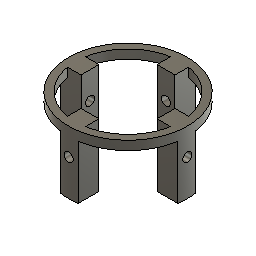
Nema17_Motor_mount_coupling_Part2 (Autodesk Fusion 360 design; units mm, degrees)
part number: 2025-04-23-20-16-13-902
Autodesk Fusion 360 part; units mm, degrees
sketch "Sketch1" plane through (0, 0, 0) normal (0, 1, 0) x (1, 0, 0)
  circle A0 centre (0, 0) radius 11
  circle A1 centre (0, 0) radius 20
  line L0 (0, 0) -> (25.4951, 0) construction
  circle A2 centre (10, 10) radius 1.5
  circle A3 centre (-10, 10) radius 1.5
  circle A4 centre (-10, -10) radius 1.5
  circle A5 centre (10, -10) radius 1.5
  dimension "d1" = 22
  dimension "d2" = 40
  dimension "d4" = 3
  dimension "d5" = 10
  dimension "d7" = 360
  constraint coincident A0.centre A1.centre
  constraint concentric A0 A1
  constraint horizontal L0
  measures "d1" diameter of A0
  measures "d2" diameter of A1
  measures "d4" diameter of A2
  measures "d5" horizontal distance of A0.centre A2.centre
extrude "Extrude1" add sketch "Sketch1" along normal blind 2
sketch "Sketch2" plane through (0, 2, 0) normal (0, 1, 0) x (-1, 0, 0)
  circle A0 centre (10, 10) radius 1.5
  circle A1 centre (10, -10) radius 1.5
  circle A2 centre (-10, -10) radius 1.5
  circle A3 centre (0, 0) radius 11
  circle A4 centre (-10, 10) radius 1.5
  circle A5 centre (0, 0) radius 20
  circle A6 centre (0, 0) radius 18
  circle A7 centre (0, 0) radius 20
  dimension "d10" = 36
  constraint concentric A3 A6
  constraint concentric A3 A7
  measures "d10" diameter of A6
extrude "Extrude2" add sketch "Sketch2" along normal blind 30 contours A5 A7
sketch "Sketch7" plane through (0, 32, 0) normal (0, 1, 0) x (-1, 0, 0)
  circle A0 centre (0, 0) radius 18
  circle A1 centre (0, 0) radius 20
  circle A2 centre (0, 0) radius 33.1
  circle A3 centre (0, 0) radius 20
  dimension "d24" = 66.2
  constraint concentric A0 A2
  constraint coincident A0.centre A1.centre
  measures "d24" diameter of A2
extrude "Extrude6" add sketch "Sketch7" against normal blind 4 contours A2
sketch "Sketch8" plane through (0, 28, 0) normal (0, -1, 0) x (1, 0, 0)
  circle A0 centre (0, 0) radius 20
  circle A1 centre (0, 0) radius 33.1
  circle A2 centre (0, 0) radius 22.5
  dimension "d31" = 45
  constraint coincident A0.centre A1.centre
  measures "d31" diameter of A2
extrude "Extrude7" add sketch "Sketch8" along normal blind 8 contours A2
sketch "Sketch9" plane through (0, 32, 0) normal (0, 1, 0) x (-1, 0, 0)
  circle A0 centre (0, 0) radius 33.1
  circle A1 centre (0, 0) radius 18
  circle A2 centre (0, 0) radius 33.1
  circle A3 centre (0, 0) radius 29.1
  line L0 (21.15, -21.15) -> (-21.15, 21.15) construction
  line L1 (-21.15, -21.15) -> (21.15, 21.15) construction
  line L2 (-5, -21.15) -> (5, -21.15)
  line L3 (5, -21.15) -> (5, -32.7202)
  line L4 (-5, -32.7202) -> (-5, -21.15)
  line L5 (-5, -21.15) -> (3.5808, -32.9057) construction
  line L6 (5, -21.15) -> (-3.5808, -32.9057) construction
  line L7 (32.7202, -5) -> (21.15, -5)
  line L8 (21.15, 5) -> (32.7202, 5)
  line L9 (21.15, -5) -> (21.15, 5)
  line L10 (5, 32.7202) -> (5, 21.15)
  line L11 (-5, 21.15) -> (-5, 32.7202)
  line L12 (5, 21.15) -> (-5, 21.15)
  line L13 (-32.7202, 5) -> (-21.15, 5)
  line L14 (-21.15, -5) -> (-32.7202, -5)
  line L15 (-21.15, 5) -> (-21.15, -5)
  point P0 (0, -28)
  dimension "d34" = 4
  dimension "d35" = 42.3
  dimension "d36" = 42.3
  constraint coincident A0.centre A1.centre
  constraint coincident L0 A0.centre
  constraint coincident L1 A0.centre
  constraint horizontal L2
  constraint perpendicular L2 L3
  constraint parallel L3 L4
  constraint coincident L5 P0
  constraint coincident L6 P0
  constraint coincident A0 L3.end
  constraint coincident A0 L4.start
  constraint coincident A0 L6.end
  constraint coincident A0 L5.end
  constraint coincident A0 L14.end
  constraint coincident A0 L13.start
  constraint coincident A0 L11.end
  constraint coincident A0 L10.start
  constraint coincident A0 L7.start
  constraint coincident A0 L8.end
  measures "d34" distance of A2 A3
  measures "d35" distance of L0.end L1.end
  measures "d36" distance of L1.start L0.end
extrude "Extrude8" add sketch "Sketch9" along normal blind 35 contours A0 A2 A3 L7 L8 | A0 A2 A3 L10 L11 | A3 L7 L8 L9 | A0 A2 A3 L3 L4 | A3 L10 L11 L12 | A3 L2 L3 L4 | A0 A2 A3 L13 L14 | A3 L13 L14 L15
extrude "Extrude9" add sketch "Sketch9" along normal blind 5 from surface at 30 contours A0 A2 A3 L8 L10 | A0 A2 A3 L3 L7 | A0 A2 A3 L11 L13 | A0 A2 A3 L4 L14
sketch "Sketch10" plane through (0, 0, 0) normal (0, 0, 1) x (1, 0, 0)
  circle A0 centre (0, 52) radius 2.5
  line L0 (33.1, 67) -> (-33.1, 67)
  line L1 (-33.1, 28) -> (33.1, 28)
  dimension "d45" = 5
  dimension "d56" = 24
  measures "d45" diameter of A0
  measures "d56" distance of A0.centre L1
extrude "Extrude10" cut sketch "Sketch10" along normal mid plane 88
sketch "Sketch11" plane through (0, 0, 0) normal (1, 0, 0) x (0, 0, -1)
  circle A0 centre (0, 52) radius 2.5
  line L0 (-33.1, 28) -> (33.1, 28)
  dimension "d49" = 5
  dimension "d55" = 24
  measures "d49" diameter of A0
  measures "d55" distance of A0.centre L0
extrude "Extrude11" cut sketch "Sketch11" along normal mid plane 90
thread "Thread1" "ISO Metric profile 40.0 M40x3 6g" major diameter 39.7645 minor diameter 36.3299 pitch 3 angle 60 modelled right hand crest width 0.4255 on face at (19.9751, 6.6667, 0.9969) from (0, 0, 0) to (0, 12.4, 0) crest through (19.8822, -0.75, 0)
extrude "Extrude12" cut sketch "Sketch9" against normal blind 50 contours A0 A2 A3 L7 L8 | A0 A2 A3 L8 L10 | A0 A2 A3 L3 L7 | A0 A2 A3 L10 L11 | A3 L2 L3 L4 L7 L8 L9 L10 L11 L12 L13 L14 L15 | A3 L7 L8 L9 | A0 A2 A3 L3 L4 | A0 A2 A3 L11 L13 | A3 L10 L11 L12 | A0 A2 A3 L4 L14 | A3 L2 L3 L4 | A0 A2 A3 L13 L14 | A3 L13 L14 L15 | A1
sketch "Sketch12" plane through (0, 32, 0) normal (0, -1, 0) x (1, 0, 0)
  line L0 (-5, 32.7202) -> (-5, 21.15)
  line L1 (-5, 21.15) -> (5, 21.15)
  line L2 (5, 21.15) -> (5, 32.7202)
  arc A0 (5, 32.7202) -> (-5, 32.7202) centre (0, 0) ccw
  circle A1 centre (0, 27.5) radius 2.5
  dimension "d59" = 5
  dimension "d60" = 27.5
  measures "d59" diameter of A1
  measures "d60" distance of A0.centre A1.centre
extrude "Extrude13" cut sketch "Sketch12" against normal blind 12 contours A1
pattern_circular "C-Pattern1" count 4 over 360 about axis through (0, 1.75, 0) along (0, 1, 0) of "Extrude13"
equation "d32 = 4 mm + 4 mm"
equation "d55 = 25 mm - 1 mm"
equation "d56 = 25 mm - 1 mm"
equation "d61 = -10.00 mm - 2 mm"
